Autodesk Fusion 360 part; units mm, degrees
note: some values were not read from the file. Set by a fixed rule: which sketch regions a step uses.
(part 41 of 59)
  spline S42 degree 5 poles (10.9662, -14.3955) (10.9662, -14.3956) (10.9663, -14.3958) (10.9664, -14.3961) (10.9666, -14.3966) (10.9669, -14.3973) (10.9672, -14.3981) (10.9676, -14.399) (10.9681, -14.4) (10.9685, -14.4011) (10.9691, -14.4023) (10.9696, -14.4036) (10.9702, -14.405) (10.9709, -14.4065) (10.9716, -14.408) (10.9724, -14.4097) (10.9731, -14.4115) (10.974, -14.4134) (10.9749, -14.4153) (10.9758, -14.4173) (10.9768, -14.4195) (10.9778, -14.4217) (10.9788, -14.424) (10.9799, -14.4263) (10.9811, -14.4288) (10.9823, -14.4313) (10.9835, -14.4339) (10.9848, -14.4366) (10.9861, -14.4394) (10.9875, -14.4423) (10.9889, -14.4452) (10.9903, -14.4482) (10.9918, -14.4513) (10.9934, -14.4544) (10.9949, -14.4577) (10.9966, -14.461) (10.9982, -14.4643) (10.9999, -14.4678) (11.0017, -14.4713) (11.0035, -14.4748) (11.0053, -14.4785) (11.0072, -14.4822) (11.0091, -14.486) (11.0111, -14.4898) (11.0131, -14.4937) (11.0151, -14.4977) (11.0172, -14.5017) (11.0193, -14.5058) (11.0215, -14.51) (11.0237, -14.5142) (11.0259, -14.5185) (11.0282, -14.5228) (11.0306, -14.5272) (11.0329, -14.5317) (11.0353, -14.5362) (11.0378, -14.5408) (11.0403, -14.5454) (11.0428, -14.5501) (11.0454, -14.5549) (11.048, -14.5597) (11.0507, -14.5645) (11.0534, -14.5694) (11.0561, -14.5744) (11.0589, -14.5794) (11.0617, -14.5845) (11.0646, -14.5896) (11.0675, -14.5948) (11.0704, -14.6) (11.0734, -14.6053) (11.0764, -14.6106) (11.0795, -14.616) (11.0826, -14.6214) (11.0857, -14.6269) (11.0889, -14.6324) (11.0921, -14.638) (11.0954, -14.6436) (11.0987, -14.6493) (11.102, -14.655) (11.1054, -14.6608) (11.1088, -14.6666) (11.1123, -14.6725) (11.1158, -14.6784) (11.1193, -14.6843) (11.1229, -14.6903) (11.1265, -14.6963) (11.1301, -14.7024) (11.1338, -14.7085) (11.1376, -14.7147) (11.1413, -14.7209) (11.1451, -14.7271) (11.149, -14.7334) (11.1529, -14.7397) (11.1568, -14.7461) (11.1608, -14.7525) (11.1648, -14.759) (11.1688, -14.7654) (11.1729, -14.772) (11.177, -14.7785) (11.1812, -14.7851) (11.1854, -14.7918) (11.1896, -14.7985) (11.1939, -14.8052) (11.1982, -14.8119) (11.2025, -14.8187) (11.2069, -14.8256) (11.2113, -14.8324) (11.2158, -14.8393) (11.2203, -14.8463) (11.2248, -14.8533) (11.2294, -14.8603) (11.234, -14.8673) (11.2387, -14.8744) (11.2434, -14.8815) (11.2481, -14.8887) (11.2529, -14.8958) (11.2577, -14.9031) (11.2625, -14.9103) (11.2674, -14.9176) (11.2723, -14.9249) (11.2773, -14.9323) (11.2823, -14.9396) (11.2873, -14.947) (11.2924, -14.9545) (11.2975, -14.962) (11.3026, -14.9695) (11.3078, -14.977) (11.313, -14.9846) (11.3183, -14.9922) (11.3235, -14.9998) (11.3289, -15.0074) (11.3342, -15.0151) (11.3396, -15.0228) (11.3451, -15.0306) (11.3506, -15.0384) (11.3561, -15.0462) (11.3616, -15.054) (11.3672, -15.0618) (11.3728, -15.0697) (11.3785, -15.0776) (11.3842, -15.0856) (11.3899, -15.0936) (11.3957, -15.1015) (11.4015, -15.1096) (11.4074, -15.1176) (11.4132, -15.1257) (11.4192, -15.1338) (11.4251, -15.1419) (11.4311, -15.1501) (11.4371, -15.1582) (11.4432, -15.1665) (11.4493, -15.1747) (11.4554, -15.1829) (11.4616, -15.1912) (11.4678, -15.1995) (11.4741, -15.2078) (11.4803, -15.2162) (11.4867, -15.2246) (11.493, -15.233) (11.4994, -15.2414) (11.5058, -15.2498) (11.5123, -15.2583) (11.5188, -15.2668) (11.5253, -15.2753) (11.5319, -15.2838) (11.5385, -15.2924) (11.5452, -15.301) (11.5518, -15.3096) (11.5585, -15.3182) (11.5653, -15.3268) (11.5721, -15.3355) (11.5789, -15.3442) (11.5858, -15.3529) (11.5927, -15.3616) (11.5996, -15.3704) (11.6065, -15.3791) (11.6135, -15.3879) (11.6206, -15.3967) (11.6276, -15.4055) (11.6348, -15.4144) (11.6419, -15.4233) (11.6491, -15.4322) (11.6563, -15.4411) (11.6635, -15.45) (11.6708, -15.4589) (11.6781, -15.4679) (11.6855, -15.4769) (11.6929, -15.4859) (11.7003, -15.4949) (11.7078, -15.5039) (11.7153, -15.513) (11.7228, -15.5221) (11.7303, -15.5312) (11.7379, -15.5403) (11.7456, -15.5494) (11.7532, -15.5585) (11.7609, -15.5677) (11.7687, -15.5769) (11.7765, -15.5861) (11.7843, -15.5953) (11.7921, -15.6045) (11.8, -15.6137) (11.8079, -15.623) (11.8158, -15.6323) (11.8238, -15.6416) (11.8318, -15.6509) (11.8399, -15.6602) (11.848, -15.6695) (11.8561, -15.6789) (11.8643, -15.6882) (11.8724, -15.6976) (11.8807, -15.707) (11.8889, -15.7164) (11.8972, -15.7259) (11.9055, -15.7353) (11.9139, -15.7447) (11.9223, -15.7542) (11.9307, -15.7637) (11.9392, -15.7732) (11.9477, -15.7827) (11.9562, -15.7922) (11.9648, -15.8018) (11.9734, -15.8113) (11.982, -15.8209) (11.9907, -15.8305) (11.9994, -15.84) (12.0081, -15.8496) (12.0169, -15.8593) (12.0257, -15.8689) (12.0345, -15.8785) (12.0434, -15.8882) (12.0523, -15.8978) (12.0613, -15.9075) (12.0702, -15.9172) (12.0792, -15.9269) (12.0883, -15.9366) (12.0973, -15.9464) (12.1065, -15.9561) (12.1156, -15.9658) (12.1248, -15.9756) (12.134, -15.9854) (12.1432, -15.9951) (12.1506, -16.003) (12.1562, -16.0089) (12.16, -16.0128) (12.1618, -16.0147) knots 0 0 0 0 0 0 0.00416667 0.00833333 0.0125 0.01666667 0.02083333 0.025 0.02916667 0.03333333 0.0375 0.04166667 0.04583333 0.05 0.05416667 0.05833333 0.0625 0.06666667 0.07083333 0.075 0.07916667 0.08333333 0.0875 0.09166667 0.09583333 0.1 0.10416667 0.10833333 0.1125 0.11666667 0.12083333 0.125 0.12916667 0.13333333 0.1375 0.14166667 0.14583333 0.15 0.15416667 0.15833333 0.1625 0.16666667 0.17083333 0.175 0.17916667 0.18333333 0.1875 0.19166667 0.19583333 0.2 0.20416667 0.20833333 0.2125 0.21666667 0.22083333 0.225 0.22916667 0.23333333 0.2375 0.24166667 0.24583333 0.25 0.25416667 0.25833333 0.2625 0.26666667 0.27083333 0.275 0.27916667 0.28333333 0.2875 0.29166667 0.29583333 0.3 0.30416667 0.30833333 0.3125 0.31666667 0.32083333 0.325 0.32916667 0.33333333 0.3375 0.34166667 0.34583333 0.35 0.35416667 0.35833333 0.3625 0.36666667 0.37083333 0.375 0.37916667 0.38333333 0.3875 0.39166667 0.39583333 0.4 0.40416667 0.40833333 0.4125 0.41666667 0.42083333 0.425 0.42916667 0.43333333 0.4375 0.44166667 0.44583333 0.45 0.45416667 0.45833333 0.4625 0.46666667 0.47083333 0.475 0.47916667 0.48333333 0.4875 0.49166667 0.49583333 0.5 0.50416667 0.50833333 0.5125 0.51666667 0.52083333 0.525 0.52916667 0.53333333 0.5375 0.54166667 0.54583333 0.55 0.55416667 0.55833333 0.5625 0.56666667 0.57083333 0.575 0.57916667 0.58333333 0.5875 0.59166667 0.59583333 0.6 0.60416667 0.60833333 0.6125 0.61666667 0.62083333 0.625 0.62916667 0.63333333 0.6375 0.64166667 0.64583333 0.65 0.65416667 0.65833333 0.6625 0.66666667 0.67083333 0.675 0.67916667 0.68333333 0.6875 0.69166667 0.69583333 0.7 0.70416667 0.70833333 0.7125 0.71666667 0.72083333 0.725 0.72916667 0.73333333 0.7375 0.74166667 0.74583333 0.75 0.75416667 0.75833333 0.7625 0.76666667 0.77083333 0.775 0.77916667 0.78333333 0.7875 0.79166667 0.79583333 0.8 0.80416667 0.80833333 0.8125 0.81666667 0.82083333 0.825 0.82916667 0.83333333 0.8375 0.84166667 0.84583333 0.85 0.85416667 0.85833333 0.8625 0.86666667 0.87083333 0.875 0.87916667 0.88333333 0.8875 0.89166667 0.89583333 0.9 0.90416667 0.90833333 0.9125 0.91666667 0.92083333 0.925 0.92916667 0.93333333 0.9375 0.94166667 0.94583333 0.95 0.95416667 0.95833333 0.9625 0.96666667 0.97083333 0.975 0.97916667 0.98333333 0.9875 0.99166667 0.99583333 1 1 1 1 1 1
  arc A43 (12.1618, -16.0147) -> (13.0527, -15.6181) centre (0, 12.5) ccw
  spline S43 degree 5 poles (13.0527, -15.6181) (13.0525, -15.6154) (13.0521, -15.61) (13.0515, -15.6019) (13.0506, -15.5911) (13.0495, -15.5777) (13.0484, -15.5644) (13.0473, -15.551) (13.0462, -15.5377) (13.0451, -15.5244) (13.0439, -15.5112) (13.0427, -15.4979) (13.0415, -15.4848) (13.0404, -15.4716) (13.0391, -15.4585) (13.0379, -15.4454) (13.0367, -15.4323) (13.0354, -15.4193) (13.0342, -15.4063) (13.0329, -15.3934) (13.0316, -15.3805) (13.0303, -15.3676) (13.029, -15.3547) (13.0276, -15.3419) (13.0263, -15.3291) (13.0249, -15.3164) (13.0236, -15.3037) (13.0222, -15.291) (13.0208, -15.2784) (13.0194, -15.2658) (13.018, -15.2532) (13.0165, -15.2406) (13.0151, -15.2281) (13.0136, -15.2157) (13.0122, -15.2032) (13.0107, -15.1908) (13.0092, -15.1785) (13.0077, -15.1661) (13.0062, -15.1539) (13.0047, -15.1416) (13.0031, -15.1294) (13.0016, -15.1172) (13, -15.105) (12.9984, -15.0929) (12.9968, -15.0809) (12.9952, -15.0688) (12.9936, -15.0568) (12.992, -15.0449) (12.9904, -15.0329) (12.9887, -15.021) (12.9871, -15.0092) (12.9854, -14.9974) (12.9838, -14.9856) (12.9821, -14.9738) (12.9804, -14.9621) (12.9787, -14.9505) (12.977, -14.9388) (12.9752, -14.9273) (12.9735, -14.9157) (12.9718, -14.9042) (12.97, -14.8927) (12.9682, -14.8813) (12.9665, -14.8699) (12.9647, -14.8585) (12.9629, -14.8472) (12.9611, -14.8359) (12.9593, -14.8247) (12.9574, -14.8135) (12.9556, -14.8023) (12.9538, -14.7912) (12.9519, -14.7801) (12.9501, -14.7691) (12.9482, -14.7581) (12.9463, -14.7471) (12.9445, -14.7362) (12.9426, -14.7253) (12.9407, -14.7145) (12.9388, -14.7037) (12.9368, -14.6929) (12.9349, -14.6822) (12.933, -14.6715) (12.9311, -14.6609) (12.9291, -14.6503) (12.9272, -14.6397) (12.9252, -14.6292) (12.9232, -14.6188) (12.9213, -14.6083) (12.9193, -14.5979) (12.9173, -14.5876) (12.9153, -14.5773) (12.9133, -14.5671) (12.9113, -14.5568) (12.9093, -14.5467) (12.9072, -14.5365) (12.9052, -14.5265) (12.9032, -14.5164) (12.9011, -14.5064) (12.8991, -14.4965) (12.8971, -14.4866) (12.895, -14.4767) (12.8929, -14.4669) (12.8909, -14.4571) (12.8888, -14.4474) (12.8867, -14.4377) (12.8847, -14.4281) (12.8826, -14.4185) (12.8805, -14.4089) (12.8784, -14.3994) (12.8763, -14.39) (12.8742, -14.3806) (12.8721, -14.3712) (12.87, -14.3619) (12.8679, -14.3526) (12.8658, -14.3434) (12.8636, -14.3342) (12.8615, -14.3251) (12.8594, -14.316) (12.8573, -14.3069) (12.8551, -14.298) (12.853, -14.289) (12.8509, -14.2801) (12.8487, -14.2713) (12.8466, -14.2625) (12.8445, -14.2537) (12.8423, -14.2451) (12.8402, -14.2364) (12.838, -14.2278) (12.8359, -14.2193) (12.8337, -14.2108) (12.8316, -14.2023) (12.8294, -14.1939) (12.8273, -14.1856) (12.8251, -14.1773) (12.823, -14.169) (12.8208, -14.1608) (12.8187, -14.1527) (12.8166, -14.1446) (12.8144, -14.1365) (12.8123, -14.1286) (12.8101, -14.1206) (12.808, -14.1127) (12.8058, -14.1049) (12.8037, -14.0971) (12.8016, -14.0894) (12.7994, -14.0817) (12.7973, -14.0741) (12.7952, -14.0665) (12.793, -14.059) (12.7909, -14.0516) (12.7888, -14.0442) (12.7867, -14.0368) (12.7845, -14.0296) (12.7824, -14.0223) (12.7803, -14.0151) (12.7782, -14.008) (12.7761, -14.0009) (12.774, -13.9939) (12.772, -13.987) (12.7699, -13.9801) (12.7678, -13.9733) (12.7657, -13.9665) (12.7637, -13.9598) (12.7616, -13.9531) (12.7596, -13.9465) (12.7575, -13.9399) (12.7555, -13.9335) (12.7534, -13.927) (12.7514, -13.9207) (12.7494, -13.9144) (12.7474, -13.9081) (12.7454, -13.9019) (12.7434, -13.8958) (12.7414, -13.8897) (12.7395, -13.8837) (12.7375, -13.8778) (12.7356, -13.8719) (12.7336, -13.8661) (12.7317, -13.8604) (12.7298, -13.8547) (12.7279, -13.8491) (12.726, -13.8435) (12.7241, -13.838) (12.7222, -13.8326) (12.7204, -13.8273) (12.7185, -13.822) (12.7167, -13.8167) (12.7149, -13.8116) (12.7131, -13.8065) (12.7113, -13.8015) (12.7095, -13.7965) (12.7077, -13.7916) (12.706, -13.7868) (12.7043, -13.782) (12.7026, -13.7774) (12.7009, -13.7728) (12.6992, -13.7682) (12.6975, -13.7638) (12.6959, -13.7594) (12.6943, -13.755) (12.6927, -13.7508) (12.6911, -13.7466) (12.6895, -13.7425) (12.688, -13.7385) (12.6864, -13.7345) (12.6849, -13.7307) (12.6834, -13.7269) (12.682, -13.7231) (12.6806, -13.7195) (12.6791, -13.7159) (12.6778, -13.7124) (12.6764, -13.709) (12.675, -13.7057) (12.6737, -13.7024) (12.6724, -13.6993) (12.6712, -13.6962) (12.6699, -13.6932) (12.6687, -13.6903) (12.6676, -13.6874) (12.6664, -13.6847) (12.6653, -13.682) (12.6642, -13.6794) (12.6631, -13.6769) (12.6621, -13.6745) (12.6611, -13.6722) (12.6602, -13.67) (12.6592, -13.6678) (12.6583, -13.6658) (12.6575, -13.6638) (12.6567, -13.6619) (12.6559, -13.6602) (12.6551, -13.6585) (12.6544, -13.6569) (12.6538, -13.6554) (12.6531, -13.654) (12.6526, -13.6527) (12.652, -13.6515) (12.6515, -13.6504) (12.651, -13.6495) (12.6506, -13.6486) (12.6503, -13.6478) (12.65, -13.6471) (12.6497, -13.6467) (12.6496, -13.6464) (12.6495, -13.6462) (12.6495, -13.6461) knots -1 -1 -1 -1 -1 -1 -0.99583333 -0.99166667 -0.9875 -0.98333333 -0.97916667 -0.975 -0.97083333 -0.96666667 -0.9625 -0.95833333 -0.95416667 -0.95 -0.94583333 -0.94166667 -0.9375 -0.93333333 -0.92916667 -0.925 -0.92083333 -0.91666667 -0.9125 -0.90833333 -0.90416667 -0.9 -0.89583333 -0.89166667 -0.8875 -0.88333333 -0.87916667 -0.875 -0.87083333 -0.86666667 -0.8625 -0.85833333 -0.85416667 -0.85 -0.84583333 -0.84166667 -0.8375 -0.83333333 -0.82916667 -0.825 -0.82083333 -0.81666667 -0.8125 -0.80833333 -0.80416667 -0.8 -0.79583333 -0.79166667 -0.7875 -0.78333333 -0.77916667 -0.775 -0.77083333 -0.76666667 -0.7625 -0.75833333 -0.75416667 -0.75 -0.74583333 -0.74166667 -0.7375 -0.73333333 -0.72916667 -0.725 -0.72083333 -0.71666667 -0.7125 -0.70833333 -0.70416667 -0.7 -0.69583333 -0.69166667 -0.6875 -0.68333333 -0.67916667 -0.675 -0.67083333 -0.66666667 -0.6625 -0.65833333 -0.65416667 -0.65 -0.64583333 -0.64166667 -0.6375 -0.63333333 -0.62916667 -0.625 -0.62083333 -0.61666667 -0.6125 -0.60833333 -0.60416667 -0.6 -0.59583333 -0.59166667 -0.5875 -0.58333333 -0.57916667 -0.575 -0.57083333 -0.56666667 -0.5625 -0.55833333 -0.55416667 -0.55 -0.54583333 -0.54166667 -0.5375 -0.53333333 -0.52916667 -0.525 -0.52083333 -0.51666667 -0.5125 -0.50833333 -0.50416667 -0.5 -0.49583333 -0.49166667 -0.4875 -0.48333333 -0.47916667 -0.475 -0.47083333 -0.46666667 -0.4625 -0.45833333 -0.45416667 -0.45 -0.44583333 -0.44166667 -0.4375 -0.43333333 -0.42916667 -0.425 -0.42083333 -0.41666667 -0.4125 -0.40833333 -0.40416667 -0.4 -0.39583333 -0.39166667 -0.3875 -0.38333333 -0.37916667 -0.375 -0.37083333 -0.36666667 -0.3625 -0.35833333 -0.35416667 -0.35 -0.34583333 -0.34166667 -0.3375 -0.33333333 -0.32916667 -0.325 -0.32083333 -0.31666667 -0.3125 -0.30833333 -0.30416667 -0.3 -0.29583333 -0.29166667 -0.2875 -0.28333333 -0.27916667 -0.275 -0.27083333 -0.26666667 -0.2625 -0.25833333 -0.25416667 -0.25 -0.24583333 -0.24166667 -0.2375 -0.23333333 -0.22916667 -0.225 -0.22083333 -0.21666667 -0.2125 -0.20833333 -0.20416667 -0.2 -0.19583333 -0.19166667 -0.1875 -0.18333333 -0.17916667 -0.175 -0.17083333 -0.16666667 -0.1625 -0.15833333 -0.15416667 -0.15 -0.14583333 -0.14166667 -0.1375 -0.13333333 -0.12916667 -0.125 -0.12083333 -0.11666667 -0.1125 -0.10833333 -0.10416667 -0.1 -0.09583333 -0.09166667 -0.0875 -0.08333333 -0.07916667 -0.075 -0.07083333 -0.06666667 -0.0625 -0.05833333 -0.05416667 -0.05 -0.04583333 -0.04166667 -0.0375 -0.03333333 -0.02916667 -0.025 -0.02083333 -0.01666667 -0.0125 -0.00833333 -0.00416667 0 0 0 0 0 0
  line L95 (12.6495, -13.6461) -> (12.6491, -13.6453)
  line L96 (12.6491, -13.6453) -> (12.5209, -13.3803)
  arc A44 (12.5209, -13.3803) -> (13.578, -12.8417) centre (0, 12.5) ccw
  line L97 (13.578, -12.8417) -> (13.7171, -13.1012)
  line L98 (13.7171, -13.1012) -> (13.7175, -13.1019)
  spline S44 degree 5 poles (13.7175, -13.1019) (13.7175, -13.102) (13.7176, -13.1022) (13.7178, -13.1025) (13.718, -13.1029) (13.7184, -13.1036) (13.7188, -13.1043) (13.7193, -13.1052) (13.7198, -13.1061) (13.7204, -13.1072) (13.721, -13.1083) (13.7217, -13.1096) (13.7225, -13.1109) (13.7233, -13.1123) (13.7242, -13.1138) (13.7251, -13.1154) (13.7261, -13.1171) (13.7271, -13.1188) (13.7282, -13.1207) (13.7293, -13.1226) (13.7305, -13.1246) (13.7317, -13.1267) (13.733, -13.1289) (13.7344, -13.1311) (13.7358, -13.1334) (13.7372, -13.1358) (13.7387, -13.1383) (13.7403, -13.1409) (13.7419, -13.1435) (13.7435, -13.1462) (13.7452, -13.1489) (13.747, -13.1518) (13.7488, -13.1547) (13.7506, -13.1577) (13.7526, -13.1607) (13.7545, -13.1638) (13.7565, -13.167) (13.7586, -13.1702) (13.7607, -13.1735) (13.7628, -13.1769) (13.765, -13.1803) (13.7673, -13.1838) (13.7696, -13.1874) (13.7719, -13.191) (13.7743, -13.1947) (13.7768, -13.1984) (13.7793, -13.2022) (13.7818, -13.206) (13.7844, -13.21) (13.787, -13.2139) (13.7897, -13.218) (13.7925, -13.222) (13.7952, -13.2262) (13.7981, -13.2304) (13.8009, -13.2346) (13.8039, -13.2389) (13.8068, -13.2432) (13.8098, -13.2476) (13.8129, -13.2521) (13.816, -13.2566) (13.8192, -13.2612) (13.8224, -13.2658) (13.8256, -13.2704) (13.8289, -13.2751) (13.8322, -13.2799) (13.8356, -13.2847) (13.839, -13.2895) (13.8425, -13.2944) (13.846, -13.2993) (13.8496, -13.3043) (13.8532, -13.3093) (13.8568, -13.3144) (13.8605, -13.3195) (13.8643, -13.3247) (13.8681, -13.3299) (13.8719, -13.3352) (13.8758, -13.3405) (13.8797, -13.3458) (13.8836, -13.3512) (13.8876, -13.3566) (13.8917, -13.3621) (13.8958, -13.3676) (13.8999, -13.3731) (13.9041, -13.3787) (13.9083, -13.3843) (13.9126, -13.39) (13.9169, -13.3957) (13.9213, -13.4014) (13.9257, -13.4072) (13.9301, -13.413) (13.9346, -13.4188) (13.9391, -13.4247) (13.9437, -13.4306) (13.9483, -13.4366) (13.9529, -13.4426) (13.9576, -13.4486) (13.9624, -13.4547) (13.9672, -13.4608) (13.972, -13.4669) (13.9769, -13.4731) (13.9818, -13.4793) (13.9867, -13.4855) (13.9917, -13.4918) (13.9967, -13.4981) (14.0018, -13.5044) (14.0069, -13.5108) (14.0121, -13.5172) (14.0173, -13.5236) (14.0225, -13.5301) (14.0278, -13.5366) (14.0332, -13.5431) (14.0385, -13.5497) (14.0439, -13.5563) (14.0494, -13.5629) (14.0549, -13.5695) (14.0604, -13.5762) (14.066, -13.5829) (14.0716, -13.5896) (14.0772, -13.5964) (14.0829, -13.6032) (14.0887, -13.61) (14.0945, -13.6168) (14.1003, -13.6237) (14.1061, -13.6306) (14.112, -13.6375) (14.118, -13.6445) (14.1239, -13.6515) (14.13, -13.6585) (14.136, -13.6655) (14.1421, -13.6726) (14.1483, -13.6796) (14.1544, -13.6868) (14.1607, -13.6939) (14.1669, -13.701) (14.1732, -13.7082) (14.1796, -13.7154) (14.1859, -13.7227) (14.1924, -13.7299) (14.1988, -13.7372) (14.2053, -13.7445) (14.2119, -13.7518) (14.2184, -13.7592) (14.225, -13.7665) (14.2317, -13.7739) (14.2384, -13.7813) (14.2451, -13.7888) (14.2519, -13.7962) (14.2587, -13.8037) (14.2656, -13.8112) (14.2724, -13.8188) (14.2794, -13.8263) (14.2863, -13.8339) (14.2933, -13.8414) (14.3004, -13.8491) (14.3075, -13.8567) (14.3146, -13.8643) (14.3217, -13.872) (14.3289, -13.8797) (14.3362, -13.8874) (14.3435, -13.8951) (14.3508, -13.9029) (14.3581, -13.9106) (14.3655, -13.9184) (14.3729, -13.9262) (14.3804, -13.934) (14.3879, -13.9419) (14.3954, -13.9497) (14.403, -13.9576) (14.4106, -13.9655) (14.4183, -13.9734) (14.426, -13.9813) (14.4337, -13.9893) (14.4415, -13.9972) (14.4493, -14.0052) (14.4571, -14.0132) (14.465, -14.0212) (14.4729, -14.0292) (14.4809, -14.0373) (14.4889, -14.0453) (14.4969, -14.0534) (14.505, -14.0615) (14.5131, -14.0696) (14.5212, -14.0777) (14.5294, -14.0858) (14.5376, -14.094) (14.5459, -14.1022) (14.5541, -14.1103) (14.5625, -14.1185) (14.5708, -14.1267) (14.5792, -14.135) (14.5877, -14.1432) (14.5961, -14.1514) (14.6046, -14.1597) (14.6132, -14.168) (14.6218, -14.1763) (14.6304, -14.1846) (14.639, -14.1929) (14.6477, -14.2012) (14.6565, -14.2096) (14.6652, -14.2179) (14.674, -14.2263) (14.6829, -14.2347) (14.6917, -14.2431) (14.7006, -14.2515) (14.7096, -14.2599) (14.7186, -14.2683) (14.7276, -14.2767) (14.7366, -14.2852) (14.7457, -14.2937) (14.7549, -14.3021) (14.764, -14.3106) (14.7732, -14.3191) (14.7824, -14.3276) (14.7917, -14.3361) (14.801, -14.3447) (14.8104, -14.3532) (14.8197, -14.3618) (14.8291, -14.3703) (14.8386, -14.3789) (14.8481, -14.3875) (14.8576, -14.3961) (14.8671, -14.4047) (14.8767, -14.4133) (14.8863, -14.4219) (14.896, -14.4305) (14.9057, -14.4392) (14.9154, -14.4478) (14.9252, -14.4565) (14.935, -14.4651) (14.9448, -14.4738) (14.9547, -14.4825) (14.9646, -14.4912) (14.9745, -14.4999) (14.9845, -14.5086) (14.9945, -14.5173) (15.0045, -14.526) (15.0146, -14.5347) (15.0247, -14.5435) (15.0349, -14.5522) (15.045, -14.561) (15.0553, -14.5697) (15.0635, -14.5767) (15.0696, -14.582) (15.0737, -14.5855) (15.0758, -14.5873) knots 0 0 0 0 0 0 0.00416667 0.00833333 0.0125 0.01666667 0.02083333 0.025 0.02916667 0.03333333 0.0375 0.04166667 0.04583333 0.05 0.05416667 0.05833333 0.0625 0.06666667 0.07083333 0.075 0.07916667 0.08333333 0.0875 0.09166667 0.09583333 0.1 0.10416667 0.10833333 0.1125 0.11666667 0.12083333 0.125 0.12916667 0.13333333 0.1375 0.14166667 0.14583333 0.15 0.15416667 0.15833333 0.1625 0.16666667 0.17083333 0.175 0.17916667 0.18333333 0.1875 0.19166667 0.19583333 0.2 0.20416667 0.20833333 0.2125 0.21666667 0.22083333 0.225 0.22916667 0.23333333 0.2375 0.24166667 0.24583333 0.25 0.25416667 0.25833333 0.2625 0.26666667 0.27083333 0.275 0.27916667 0.28333333 0.2875 0.29166667 0.29583333 0.3 0.30416667 0.30833333 0.3125 0.31666667 0.32083333 0.325 0.32916667 0.33333333 0.3375 0.34166667 0.34583333 0.35 0.35416667 0.35833333 0.3625 0.36666667 0.37083333 0.375 0.37916667 0.38333333 0.3875 0.39166667 0.39583333 0.4 0.40416667 0.40833333 0.4125 0.41666667 0.42083333 0.425 0.42916667 0.43333333 0.4375 0.44166667 0.44583333 0.45 0.45416667 0.45833333 0.4625 0.46666667 0.47083333 0.475 0.47916667 0.48333333 0.4875 0.49166667 0.49583333 0.5 0.50416667 0.50833333 0.5125 0.51666667 0.52083333 0.525 0.52916667 0.53333333 0.5375 0.54166667 0.54583333 0.55 0.55416667 0.55833333 0.5625 0.56666667 0.57083333 0.575 0.57916667 0.58333333 0.5875 0.59166667 0.59583333 0.6 0.60416667 0.60833333 0.6125 0.61666667 0.62083333 0.625 0.62916667 0.63333333 0.6375 0.64166667 0.64583333 0.65 0.65416667 0.65833333 0.6625 0.66666667 0.67083333 0.675 0.67916667 0.68333333 0.6875 0.69166667 0.69583333 0.7 0.70416667 0.70833333 0.7125 0.71666667 0.72083333 0.725 0.72916667 0.73333333 0.7375 0.74166667 0.74583333 0.75 0.75416667 0.75833333 0.7625 0.76666667 0.77083333 0.775 0.77916667 0.78333333 0.7875 0.79166667 0.79583333 0.8 0.80416667 0.80833333 0.8125 0.81666667 0.82083333 0.825 0.82916667 0.83333333 0.8375 0.84166667 0.84583333 0.85 0.85416667 0.85833333 0.8625 0.86666667 0.87083333 0.875 0.87916667 0.88333333 0.8875 0.89166667 0.89583333 0.9 0.90416667 0.90833333 0.9125 0.91666667 0.92083333 0.925 0.92916667 0.93333333 0.9375 0.94166667 0.94583333 0.95 0.95416667 0.95833333 0.9625 0.96666667 0.97083333 0.975 0.97916667 0.98333333 0.9875 0.99166667 0.99583333 1 1 1 1 1 1
  arc A45 (15.0758, -14.5873) -> (15.9204, -14.0997) centre (0, 12.5) ccw
  spline S45 degree 5 poles (15.9204, -14.0997) (15.9199, -14.097) (15.9189, -14.0917) (15.9174, -14.0837) (15.9154, -14.0731) (15.913, -14.0599) (15.9105, -14.0467) (15.908, -14.0335) (15.9055, -14.0204) (15.9029, -14.0073) (15.9004, -13.9943) (15.8979, -13.9812) (15.8953, -13.9682) (15.8927, -13.9553) (15.8902, -13.9424) (15.8876, -13.9295) (15.885, -13.9166) (15.8824, -13.9038) (15.8798, -13.891) (15.8771, -13.8783) (15.8745, -13.8656) (15.8719, -13.8529) (15.8692, -13.8403) (15.8666, -13.8276) (15.8639, -13.8151) (15.8612, -13.8025) (15.8585, -13.79) (15.8558, -13.7776) (15.8531, -13.7651) (15.8504, -13.7528) (15.8477, -13.7404) (15.8449, -13.7281) (15.8422, -13.7158) (15.8394, -13.7035) (15.8367, -13.6913) (15.8339, -13.6792) (15.8311, -13.667) (15.8283, -13.6549) (15.8255, -13.6428) (15.8227, -13.6308) (15.8199, -13.6188) (15.8171, -13.6069) (15.8143, -13.595) (15.8115, -13.5831) (15.8086, -13.5712) (15.8058, -13.5594) (15.8029, -13.5477) (15.8001, -13.5359) (15.7972, -13.5242) (15.7943, -13.5126) (15.7914, -13.501) (15.7886, -13.4894) (15.7857, -13.4778) (15.7828, -13.4663) (15.7798, -13.4549) (15.7769, -13.4435) (15.774, -13.4321) (15.7711, -13.4207) (15.7682, -13.4094) (15.7652, -13.3982) (15.7623, -13.3869) (15.7593, -13.3757) (15.7564, -13.3646) (15.7534, -13.3535) (15.7504, -13.3424) (15.7475, -13.3314) (15.7445, -13.3204) (15.7415, -13.3094) (15.7385, -13.2985) (15.7355, -13.2877) (15.7325, -13.2768) (15.7295, -13.266) (15.7265, -13.2553) (15.7235, -13.2446) (15.7205, -13.2339) (15.7175, -13.2233) (15.7145, -13.2127) (15.7114, -13.2022) (15.7084, -13.1917) (15.7054, -13.1812) (15.7023, -13.1708) (15.6993, -13.1604) (15.6963, -13.1501) (15.6932, -13.1398) (15.6902, -13.1296) (15.6871, -13.1194) (15.6841, -13.1092) (15.681, -13.0991) (15.6779, -13.089) (15.6749, -13.079) (15.6718, -13.069) (15.6688, -13.059) (15.6657, -13.0491) (15.6626, -13.0393) (15.6596, -13.0294) (15.6565, -13.0197) (15.6534, -13.0099) (15.6503, -13.0003) (15.6473, -12.9906) (15.6442, -12.981) (15.6411, -12.9715) (15.638, -12.962) (15.635, -12.9525) (15.6319, -12.9431) (15.6288, -12.9337) (15.6257, -12.9244) (15.6227, -12.9151) (15.6196, -12.9059) (15.6165, -12.8967) (15.6134, -12.8876) (15.6104, -12.8785) (15.6073, -12.8694) (15.6042, -12.8604) (15.6012, -12.8515) (15.5981, -12.8426) (15.595, -12.8337) (15.592, -12.8249) (15.5889, -12.8161) (15.5859, -12.8074) (15.5828, -12.7988) (15.5798, -12.7901) (15.5767, -12.7816) (15.5737, -12.7731) (15.5706, -12.7646) (15.5676, -12.7562) (15.5645, -12.7478) (15.5615, -12.7394) (15.5585, -12.7312) (15.5555, -12.7229) (15.5524, -12.7148) (15.5494, -12.7066) (15.5464, -12.6986) (15.5434, -12.6905) (15.5404, -12.6826) (15.5374, -12.6746) (15.5344, -12.6668) (15.5315, -12.6589) (15.5285, -12.6512) (15.5255, -12.6434) (15.5226, -12.6358) (15.5196, -12.6282) (15.5166, -12.6206) (15.5137, -12.6131) (15.5108, -12.6056) (15.5078, -12.5982) (15.5049, -12.5909) (15.502, -12.5836) (15.4991, -12.5763) (15.4962, -12.5691) (15.4933, -12.562) (15.4905, -12.5549) (15.4876, -12.5479) (15.4848, -12.5409) (15.4819, -12.534) (15.4791, -12.5271) (15.4762, -12.5203) (15.4734, -12.5136) (15.4706, -12.5069) (15.4678, -12.5002) (15.4651, -12.4936) (15.4623, -12.4871) (15.4595, -12.4806) (15.4568, -12.4742) (15.4541, -12.4679) (15.4514, -12.4616) (15.4486, -12.4553) (15.446, -12.4492) (15.4433, -12.443) (15.4406, -12.437) (15.438, -12.431) (15.4353, -12.425) (15.4327, -12.4192) (15.4301, -12.4133) (15.4275, -12.4076) (15.425, -12.4019) (15.4224, -12.3962) (15.4199, -12.3907) (15.4174, -12.3852) (15.4149, -12.3797) (15.4124, -12.3743) (15.4099, -12.369) (15.4075, -12.3637) (15.405, -12.3585) (15.4026, -12.3534) (15.4002, -12.3483) (15.3979, -12.3433) (15.3955, -12.3384) (15.3932, -12.3335) (15.3909, -12.3287) (15.3886, -12.3239) (15.3863, -12.3193) (15.3841, -12.3147) (15.3819, -12.3101) (15.3797, -12.3056) (15.3775, -12.3012) (15.3754, -12.2969) (15.3733, -12.2926) (15.3712, -12.2884) (15.3691, -12.2843) (15.3671, -12.2802) (15.3651, -12.2763) (15.3631, -12.2723) (15.3611, -12.2685) (15.3592, -12.2647) (15.3573, -12.261) (15.3554, -12.2574) (15.3536, -12.2539) (15.3518, -12.2504) (15.35, -12.247) (15.3482, -12.2437) (15.3465, -12.2404) (15.3449, -12.2372) (15.3432, -12.2341) (15.3416, -12.2311) (15.34, -12.2282) (15.3385, -12.2253) (15.337, -12.2225) (15.3355, -12.2198) (15.3341, -12.2172) (15.3327, -12.2147) (15.3313, -12.2122) (15.33, -12.2099) (15.3287, -12.2076) (15.3275, -12.2054) (15.3263, -12.2033) (15.3252, -12.2012) (15.3241, -12.1993) (15.323, -12.1974) (15.322, -12.1956) (15.321, -12.194) (15.3201, -12.1924) (15.3193, -12.1909) (15.3184, -12.1895) (15.3177, -12.1881) (15.3169, -12.1869) (15.3163, -12.1858) (15.3157, -12.1848) (15.3151, -12.1838) (15.3146, -12.183) (15.3142, -12.1822) (15.3138, -12.1816) (15.3135, -12.1812) (15.3133, -12.1809) (15.3132, -12.1807) (15.3132, -12.1806) knots -1 -1 -1 -1 -1 -1 -0.99583333 -0.99166667 -0.9875 -0.98333333 -0.97916667 -0.975 -0.97083333 -0.96666667 -0.9625 -0.95833333 -0.95416667 -0.95 -0.94583333 -0.94166667 -0.9375 -0.93333333 -0.92916667 -0.925 -0.92083333 -0.91666667 -0.9125 -0.90833333 -0.90416667 -0.9 -0.89583333 -0.89166667 -0.8875 -0.88333333 -0.87916667 -0.875 -0.87083333 -0.86666667 -0.8625 -0.85833333 -0.85416667 -0.85 -0.84583333 -0.84166667 -0.8375 -0.83333333 -0.82916667 -0.825 -0.82083333 -0.81666667 -0.8125 -0.80833333 -0.80416667 -0.8 -0.79583333 -0.79166667 -0.7875 -0.78333333 -0.77916667 -0.775 -0.77083333 -0.76666667 -0.7625 -0.75833333 -0.75416667 -0.75 -0.74583333 -0.74166667 -0.7375 -0.73333333 -0.72916667 -0.725 -0.72083333 -0.71666667 -0.7125 -0.70833333 -0.70416667 -0.7 -0.69583333 -0.69166667 -0.6875 -0.68333333 -0.67916667 -0.675 -0.67083333 -0.66666667 -0.6625 -0.65833333 -0.65416667 -0.65 -0.64583333 -0.64166667 -0.6375 -0.63333333 -0.62916667 -0.625 -0.62083333 -0.61666667 -0.6125 -0.60833333 -0.60416667 -0.6 -0.59583333 -0.59166667 -0.5875 -0.58333333 -0.57916667 -0.575 -0.57083333 -0.56666667 -0.5625 -0.55833333 -0.55416667 -0.55 -0.54583333 -0.54166667 -0.5375 -0.53333333 -0.52916667 -0.525 -0.52083333 -0.51666667 -0.5125 -0.50833333 -0.50416667 -0.5 -0.49583333 -0.49166667 -0.4875 -0.48333333 -0.47916667 -0.475 -0.47083333 -0.46666667 -0.4625 -0.45833333 -0.45416667 -0.45 -0.44583333 -0.44166667 -0.4375 -0.43333333 -0.42916667 -0.425 -0.42083333 -0.41666667 -0.4125 -0.40833333 -0.40416667 -0.4 -0.39583333 -0.39166667 -0.3875 -0.38333333 -0.37916667 -0.375 -0.37083333 -0.36666667 -0.3625 -0.35833333 -0.35416667 -0.35 -0.34583333 -0.34166667 -0.3375 -0.33333333 -0.32916667 -0.325 -0.32083333 -0.31666667 -0.3125 -0.30833333 -0.30416667 -0.3 -0.29583333 -0.29166667 -0.2875 -0.28333333 -0.27916667 -0.275 -0.27083333 -0.26666667 -0.2625 -0.25833333 -0.25416667 -0.25 -0.24583333 -0.24166667 -0.2375 -0.23333333 -0.22916667 -0.225 -0.22083333 -0.21666667 -0.2125 -0.20833333 -0.20416667 -0.2 -0.19583333 -0.19166667 -0.1875 -0.18333333 -0.17916667 -0.175 -0.17083333 -0.16666667 -0.1625 -0.15833333 -0.15416667 -0.15 -0.14583333 -0.14166667 -0.1375 -0.13333333 -0.12916667 -0.125 -0.12083333 -0.11666667 -0.1125 -0.10833333 -0.10416667 -0.1 -0.09583333 -0.09166667 -0.0875 -0.08333333 -0.07916667 -0.075 -0.07083333 -0.06666667 -0.0625 -0.05833333 -0.05416667 -0.05 -0.04583333 -0.04166667 -0.0375 -0.03333333 -0.02916667 -0.025 -0.02083333 -0.01666667 -0.0125 -0.00833333 -0.00416667 0 0 0 0 0 0
  line L99 (15.3132, -12.1806) -> (15.3128, -12.1799)
  line L100 (15.3128, -12.1799) -> (15.1575, -11.9297)
  arc A46 (15.1575, -11.9297) -> (16.1526, -11.2836) centre (0, 12.5) ccw
  line L101 (16.1526, -11.2836) -> (16.318, -11.5271)
  line L102 (16.318, -11.5271) -> (16.3184, -11.5278)
  spline S46 degree 5 poles (16.3184, -11.5278) (16.3185, -11.5279) (16.3186, -11.5281) (16.3188, -11.5283) (16.3191, -11.5287) (16.3195, -11.5294) (16.32, -11.5301) (16.3206, -11.5309) (16.3212, -11.5317) (16.3219, -11.5327) (16.3227, -11.5338) (16.3235, -11.535) (16.3244, -11.5362) (16.3253, -11.5375) (16.3263, -11.5389) (16.3274, -11.5404) (16.3286, -11.542) (16.3298, -11.5436) (16.331, -11.5453) (16.3324, -11.5471) (16.3338, -11.549) (16.3352, -11.551) (16.3367, -11.553) (16.3383, -11.5551) (16.3399, -11.5572) (16.3416, -11.5595) (16.3434, -11.5618) (16.3452, -11.5641) (16.3471, -11.5666) (16.349, -11.5691) (16.351, -11.5717) (16.353, -11.5743) (16.3551, -11.577) (16.3573, -11.5798) (16.3595, -11.5826) (16.3618, -11.5855) (16.3641, -11.5884) (16.3665, -11.5914) (16.3689, -11.5945) (16.3714, -11.5976) (16.374, -11.6008) (16.3766, -11.604) (16.3792, -11.6073) (16.3819, -11.6107) (16.3847, -11.6141) (16.3875, -11.6176) (16.3904, -11.6211) (16.3933, -11.6246) (16.3963, -11.6283) (16.3994, -11.6319) (16.4024, -11.6356) (16.4056, -11.6394) (16.4088, -11.6432) (16.412, -11.6471) (16.4153, -11.651) (16.4187, -11.655) (16.4221, -11.659) (16.4256, -11.6631) (16.4291, -11.6672) (16.4326, -11.6713) (16.4362, -11.6755) (16.4399, -11.6798) (16.4436, -11.6841) (16.4474, -11.6884) (16.4512, -11.6928) (16.455, -11.6972) (16.459, -11.7017) (16.4629, -11.7062) (16.4669, -11.7107) (16.471, -11.7153) (16.4751, -11.7199) (16.4793, -11.7246) (16.4835, -11.7293) (16.4877, -11.734) (16.492, -11.7388) (16.4964, -11.7436) (16.5008, -11.7485) (16.5053, -11.7534) (16.5098, -11.7583) (16.5143, -11.7633) (16.5189, -11.7683) (16.5236, -11.7733) (16.5282, -11.7784) (16.533, -11.7835) (16.5378, -11.7887) (16.5426, -11.7939) (16.5475, -11.7991) (16.5524, -11.8043) (16.5574, -11.8096) (16.5624, -11.8149) (16.5675, -11.8203) (16.5726, -11.8257) (16.5778, -11.8311) (16.583, -11.8365) (16.5882, -11.842) (16.5935, -11.8475) (16.5989, -11.853) (16.6043, -11.8586) (16.6097, -11.8642) (16.6152, -11.8698) (16.6207, -11.8755) (16.6263, -11.8812) (16.6319, -11.8869) (16.6376, -11.8926) (16.6433, -11.8984) (16.6491, -11.9042) (16.6549, -11.91) (16.6607, -11.9159) (16.6666, -11.9218) (16.6725, -11.9277) (16.6785, -11.9336) (16.6845, -11.9395) (16.6906, -11.9455) (16.6967, -11.9515) (16.7029, -11.9576) (16.7091, -11.9636) (16.7153, -11.9697) (16.7216, -11.9758) (16.7279, -11.982) (16.7343, -11.9881) (16.7407, -11.9943) (16.7472, -12.0005) (16.7537, -12.0067) (16.7602, -12.013) (16.7668, -12.0192) (16.7735, -12.0255) (16.7801, -12.0319) (16.7869, -12.0382) (16.7936, -12.0446) (16.8004, -12.0509) (16.8073, -12.0573) (16.8142, -12.0638) (16.8211, -12.0702) (16.8281, -12.0767) (16.8351, -12.0831) (16.8421, -12.0897) (16.8492, -12.0962) (16.8564, -12.1027) (16.8636, -12.1093) (16.8708, -12.1159) (16.8781, -12.1225) (16.8854, -12.1291) (16.8927, -12.1357) (16.9001, -12.1424) (16.9075, -12.1491) (16.915, -12.1558) (16.9225, -12.1625) (16.9301, -12.1692) (16.9377, -12.1759) (16.9453, -12.1827) (16.953, -12.1895) (16.9607, -12.1963) (16.9685, -12.2031) (16.9763, -12.2099) (16.9841, -12.2168) (16.992, -12.2236) (16.9999, -12.2305) (17.0079, -12.2374) (17.0159, -12.2443) (17.0239, -12.2512) (17.032, -12.2582) (17.0401, -12.2651) (17.0483, -12.2721) (17.0565, -12.2791) (17.0647, -12.2861) (17.073, -12.2931) (17.0813, -12.3001) (17.0897, -12.3071) (17.0981, -12.3142) (17.1065, -12.3212) (17.115, -12.3283) (17.1235, -12.3354) (17.1321, -12.3425) (17.1407, -12.3496) (17.1493, -12.3568) (17.158, -12.3639) (17.1667, -12.3711) (17.1754, -12.3782) (17.1842, -12.3854) (17.1931, -12.3926) (17.2019, -12.3998) (17.2108, -12.407) (17.2198, -12.4142) (17.2288, -12.4215) (17.2378, -12.4287) (17.2469, -12.436) (17.2559, -12.4432) (17.2651, -12.4505) (17.2743, -12.4578) (17.2835, -12.4651) (17.2927, -12.4724) (17.302, -12.4797) (17.3113, -12.4871) (17.3207, -12.4944) (17.3301, -12.5017) (17.3395, -12.5091) (17.349, -12.5165) (17.3585, -12.5238) (17.3681, -12.5312) (17.3777, -12.5386) (17.3873, -12.546) (17.397, -12.5534) (17.4067, -12.5609) (17.4164, -12.5683) (17.4262, -12.5757) (17.436, -12.5832) (17.4458, -12.5906) (17.4557, -12.5981) (17.4657, -12.6055) (17.4756, -12.613) (17.4856, -12.6205) (17.4956, -12.628) (17.5057, -12.6355) (17.5158, -12.643) (17.526, -12.6505) (17.5361, -12.658) (17.5464, -12.6655) (17.5566, -12.6731) (17.5669, -12.6806) (17.5772, -12.6881) (17.5876, -12.6957) (17.598, -12.7032) (17.6084, -12.7108) (17.6189, -12.7184) (17.6294, -12.7259) (17.6399, -12.7335) (17.6505, -12.7411) (17.6611, -12.7487) (17.6718, -12.7563) (17.6825, -12.7639) (17.6932, -12.7715) (17.7039, -12.7791) (17.7147, -12.7867) (17.7256, -12.7943) (17.7364, -12.8019) (17.7473, -12.8096) (17.7583, -12.8172) (17.7692, -12.8248) (17.7802, -12.8325) (17.7913, -12.8401) (17.8023, -12.8477) (17.8112, -12.8539) (17.8179, -12.8584) (17.8224, -12.8615) (17.8246, -12.863) knots 0 0 0 0 0 0 0.00416667 0.00833333 0.0125 0.01666667 0.02083333 0.025 0.02916667 0.03333333 0.0375 0.04166667 0.04583333 0.05 0.05416667 0.05833333 0.0625 0.06666667 0.07083333 0.075 0.07916667 0.08333333 0.0875 0.09166667 0.09583333 0.1 0.10416667 0.10833333 0.1125 0.11666667 0.12083333 0.125 0.12916667 0.13333333 0.1375 0.14166667 0.14583333 0.15 0.15416667 0.15833333 0.1625 0.16666667 0.17083333 0.175 0.17916667 0.18333333 0.1875 0.19166667 0.19583333 0.2 0.20416667 0.20833333 0.2125 0.21666667 0.22083333 0.225 0.22916667 0.23333333 0.2375 0.24166667 0.24583333 0.25 0.25416667 0.25833333 0.2625 0.26666667 0.27083333 0.275 0.27916667 0.28333333 0.2875 0.29166667 0.29583333 0.3 0.30416667 0.30833333 0.3125 0.31666667 0.32083333 0.325 0.32916667 0.33333333 0.3375 0.34166667 0.34583333 0.35 0.35416667 0.35833333 0.3625 0.36666667 0.37083333 0.375 0.37916667 0.38333333 0.3875 0.39166667 0.39583333 0.4 0.40416667 0.40833333 0.4125 0.41666667 0.42083333 0.425 0.42916667 0.43333333 0.4375 0.44166667 0.44583333 0.45 0.45416667 0.45833333 0.4625 0.46666667 0.47083333 0.475 0.47916667 0.48333333 0.4875 0.49166667 0.49583333 0.5 0.50416667 0.50833333 0.5125 0.51666667 0.52083333 0.525 0.52916667 0.53333333 0.5375 0.54166667 0.54583333 0.55 0.55416667 0.55833333 0.5625 0.56666667 0.57083333 0.575 0.57916667 0.58333333 0.5875 0.59166667 0.59583333 0.6 0.60416667 0.60833333 0.6125 0.61666667 0.62083333 0.625 0.62916667 0.63333333 0.6375 0.64166667 0.64583333 0.65 0.65416667 0.65833333 0.6625 0.66666667 0.67083333 0.675 0.67916667 0.68333333 0.6875 0.69166667 0.69583333 0.7 0.70416667 0.70833333 0.7125 0.71666667 0.72083333 0.725 0.72916667 0.73333333 0.7375 0.74166667 0.74583333 0.75 0.75416667 0.75833333 0.7625 0.76666667 0.77083333 0.775 0.77916667 0.78333333 0.7875 0.79166667 0.79583333 0.8 0.80416667 0.80833333 0.8125 0.81666667 0.82083333 0.825 0.82916667 0.83333333 0.8375 0.84166667 0.84583333 0.85 0.85416667 0.85833333 0.8625 0.86666667 0.87083333 0.875 0.87916667 0.88333333 0.8875 0.89166667 0.89583333 0.9 0.90416667 0.90833333 0.9125 0.91666667 0.92083333 0.925 0.92916667 0.93333333 0.9375 0.94166667 0.94583333 0.95 0.95416667 0.95833333 0.9625 0.96666667 0.97083333 0.975 0.97916667 0.98333333 0.9875 0.99166667 0.99583333 1 1 1 1 1 1
  arc A47 (17.8246, -12.863) -> (18.6136, -12.2898) centre (0, 12.5) ccw
  spline S47 degree 5 poles (18.6136, -12.2898) (18.6128, -12.2872) (18.6113, -12.282) (18.609, -12.2743) (18.6059, -12.2639) (18.6021, -12.251) (18.5982, -12.2382) (18.5943, -12.2253) (18.5905, -12.2125) (18.5866, -12.1998) (18.5827, -12.1871) (18.5788, -12.1744) (18.5749, -12.1617) (18.571, -12.1491) (18.5671, -12.1365) (18.5632, -12.124) (18.5593, -12.1115) (18.5553, -12.099) (18.5514, -12.0866) (18.5475, -12.0742) (18.5435, -12.0618) (18.5395, -12.0495) (18.5356, -12.0372) (18.5316, -12.0249) (18.5277, -12.0127) (18.5237, -12.0005) (18.5197, -11.9884) (18.5157, -11.9762) (18.5117, -11.9642) (18.5077, -11.9521) (18.5037, -11.9401) (18.4997, -11.9281) (18.4957, -11.9162) (18.4917, -11.9043) (18.4877, -11.8925) (18.4836, -11.8806) (18.4796, -11.8689) (18.4756, -11.8571) (18.4715, -11.8454) (18.4675, -11.8337) (18.4634, -11.8221) (18.4594, -11.8105) (18.4553, -11.799) (18.4513, -11.7874) (18.4472, -11.776) (18.4431, -11.7645) (18.4391, -11.7531) (18.435, -11.7417) (18.4309, -11.7304) (18.4269, -11.7191) (18.4228, -11.7079) (18.4187, -11.6967) (18.4146, -11.6855) (18.4105, -11.6744) (18.4064, -11.6633) (18.4023, -11.6522) (18.3982, -11.6412) (18.3941, -11.6302) (18.39, -11.6193) (18.3859, -11.6084) (18.3818, -11.5975) (18.3777, -11.5867) (18.3736, -11.5759) (18.3695, -11.5652) (18.3654, -11.5545) (18.3613, -11.5438) (18.3572, -11.5332) (18.3531, -11.5226) (18.349, -11.5121) (18.3449, -11.5016) (18.3408, -11.4911) (18.3366, -11.4807) (18.3325, -11.4703) (18.3284, -11.46) (18.3243, -11.4497) (18.3202, -11.4395) (18.3161, -11.4292) (18.312, -11.4191) (18.3079, -11.409) (18.3038, -11.3989) (18.2996, -11.3888) (18.2955, -11.3788) (18.2914, -11.3689) (18.2873, -11.359) (18.2832, -11.3491) (18.2791, -11.3393) (18.275, -11.3295) (18.2709, -11.3197) (18.2668, -11.31) (18.2627, -11.3004) (18.2587, -11.2907) (18.2546, -11.2812) (18.2505, -11.2716) (18.2464, -11.2622) (18.2423, -11.2527) (18.2383, -11.2433) (18.2342, -11.234) (18.2301, -11.2247) (18.226, -11.2154) (18.222, -11.2062) (18.2179, -11.197) (18.2139, -11.1879) (18.2098, -11.1788) (18.2058, -11.1697) (18.2018, -11.1607) (18.1977, -11.1518) (18.1937, -11.1429) (18.1897, -11.134) (18.1857, -11.1252) (18.1816, -11.1165) (18.1776, -11.1077) (18.1736, -11.0991) (18.1696, -11.0904) (18.1657, -11.0818) (18.1617, -11.0733) (18.1577, -11.0648) (18.1537, -11.0564) (18.1498, -11.048) (18.1458, -11.0396) (18.1419, -11.0313) (18.1379, -11.0231) (18.134, -11.0149) (18.1301, -11.0067) (18.1262, -10.9986) (18.1223, -10.9905) (18.1184, -10.9825) (18.1145, -10.9746) (18.1106, -10.9666) (18.1068, -10.9588) (18.1029, -10.951) (18.0991, -10.9432) (18.0952, -10.9355) (18.0914, -10.9278) (18.0876, -10.9202) (18.0838, -10.9126) (18.08, -10.9051) (18.0762, -10.8976) (18.0724, -10.8902) (18.0687, -10.8828) (18.0649, -10.8755) (18.0612, -10.8683) (18.0575, -10.861) (18.0538, -10.8539) (18.0501, -10.8468) (18.0464, -10.8397) (18.0427, -10.8327) (18.039, -10.8257) (18.0354, -10.8188) (18.0318, -10.812) (18.0282, -10.8052) (18.0246, -10.7984) (18.021, -10.7918) (18.0174, -10.7851) (18.0139, -10.7785) (18.0103, -10.772) (18.0068, -10.7655) (18.0033, -10.7591) (17.9998, -10.7527) (17.9963, -10.7464) (17.9929, -10.7402) (17.9895, -10.734) (17.986, -10.7278) (17.9826, -10.7217) (17.9793, -10.7157) (17.9759, -10.7097) (17.9726, -10.7038) (17.9692, -10.6979) (17.9659, -10.6921) (17.9627, -10.6864) (17.9594, -10.6807) (17.9562, -10.6751) (17.9529, -10.6695) (17.9497, -10.664) (17.9466, -10.6585) (17.9434, -10.6531) (17.9403, -10.6478) (17.9372, -10.6425) (17.9341, -10.6373) (17.931, -10.6321) (17.928, -10.627) (17.925, -10.622) (17.922, -10.617) (17.9191, -10.6121) (17.9161, -10.6072) (17.9132, -10.6024) (17.9103, -10.5977) (17.9075, -10.593) (17.9047, -10.5884) (17.9019, -10.5839) (17.8991, -10.5794) (17.8964, -10.575) (17.8937, -10.5706) (17.891, -10.5664) (17.8883, -10.5621) (17.8857, -10.558) (17.8831, -10.5539) (17.8806, -10.5499) (17.8781, -10.5459) (17.8756, -10.542) (17.8731, -10.5382) (17.8707, -10.5344) (17.8683, -10.5308) (17.866, -10.5271) (17.8637, -10.5236) (17.8614, -10.5201) (17.8592, -10.5167) (17.857, -10.5134) (17.8548, -10.5101) (17.8527, -10.5069) (17.8506, -10.5038) (17.8485, -10.5007) (17.8465, -10.4978) (17.8446, -10.4948) (17.8427, -10.492) (17.8408, -10.4893) (17.8389, -10.4866) (17.8372, -10.484) (17.8354, -10.4814) (17.8337, -10.479) (17.8321, -10.4766) (17.8305, -10.4743) (17.8289, -10.4721) (17.8274, -10.4699) (17.826, -10.4679) (17.8246, -10.4659) (17.8232, -10.464) (17.8219, -10.4622) (17.8207, -10.4604) (17.8195, -10.4588) (17.8183, -10.4572) (17.8172, -10.4557) (17.8162, -10.4543) (17.8153, -10.453) (17.8144, -10.4518) (17.8135, -10.4506) (17.8127, -10.4496) (17.812, -10.4486) (17.8114, -10.4477) (17.8108, -10.4469) (17.8103, -10.4463) (17.8098, -10.4457) (17.8095, -10.4453) (17.8093, -10.445) (17.8092, -10.4448) (17.8091, -10.4448) knots -1 -1 -1 -1 -1 -1 -0.99583333 -0.99166667 -0.9875 -0.98333333 -0.97916667 -0.975 -0.97083333 -0.96666667 -0.9625 -0.95833333 -0.95416667 -0.95 -0.94583333 -0.94166667 -0.9375 -0.93333333 -0.92916667 -0.925 -0.92083333 -0.91666667 -0.9125 -0.90833333 -0.90416667 -0.9 -0.89583333 -0.89166667 -0.8875 -0.88333333 -0.87916667 -0.875 -0.87083333 -0.86666667 -0.8625 -0.85833333 -0.85416667 -0.85 -0.84583333 -0.84166667 -0.8375 -0.83333333 -0.82916667 -0.825 -0.82083333 -0.81666667 -0.8125 -0.80833333 -0.80416667 -0.8 -0.79583333 -0.79166667 -0.7875 -0.78333333 -0.77916667 -0.775 -0.77083333 -0.76666667 -0.7625 -0.75833333 -0.75416667 -0.75 -0.74583333 -0.74166667 -0.7375 -0.73333333 -0.72916667 -0.725 -0.72083333 -0.71666667 -0.7125 -0.70833333 -0.70416667 -0.7 -0.69583333 -0.69166667 -0.6875 -0.68333333 -0.67916667 -0.675 -0.67083333 -0.66666667 -0.6625 -0.65833333 -0.65416667 -0.65 -0.64583333 -0.64166667 -0.6375 -0.63333333 -0.62916667 -0.625 -0.62083333 -0.61666667 -0.6125 -0.60833333 -0.60416667 -0.6 -0.59583333 -0.59166667 -0.5875 -0.58333333 -0.57916667 -0.575 -0.57083333 -0.56666667 -0.5625 -0.55833333 -0.55416667 -0.55 -0.54583333 -0.54166667 -0.5375 -0.53333333 -0.52916667 -0.525 -0.52083333 -0.51666667 -0.5125 -0.50833333 -0.50416667 -0.5 -0.49583333 -0.49166667 -0.4875 -0.48333333 -0.47916667 -0.475 -0.47083333 -0.46666667 -0.4625 -0.45833333 -0.45416667 -0.45 -0.44583333 -0.44166667 -0.4375 -0.43333333 -0.42916667 -0.425 -0.42083333 -0.41666667 -0.4125 -0.40833333 -0.40416667 -0.4 -0.39583333 -0.39166667 -0.3875 -0.38333333 -0.37916667 -0.375 -0.37083333 -0.36666667 -0.3625 -0.35833333 -0.35416667 -0.35 -0.34583333 -0.34166667 -0.3375 -0.33333333 -0.32916667 -0.325 -0.32083333 -0.31666667 -0.3125 -0.30833333 -0.30416667 -0.3 -0.29583333 -0.29166667 -0.2875 -0.28333333 -0.27916667 -0.275 -0.27083333 -0.26666667 -0.2625 -0.25833333 -0.25416667 -0.25 -0.24583333 -0.24166667 -0.2375 -0.23333333 -0.22916667 -0.225 -0.22083333 -0.21666667 -0.2125 -0.20833333 -0.20416667 -0.2 -0.19583333 -0.19166667 -0.1875 -0.18333333 -0.17916667 -0.175 -0.17083333 -0.16666667 -0.1625 -0.15833333 -0.15416667 -0.15 -0.14583333 -0.14166667 -0.1375 -0.13333333 -0.12916667 -0.125 -0.12083333 -0.11666667 -0.1125 -0.10833333 -0.10416667 -0.1 -0.09583333 -0.09166667 -0.0875 -0.08333333 -0.07916667 -0.075 -0.07083333 -0.06666667 -0.0625 -0.05833333 -0.05416667 -0.05 -0.04583333 -0.04166667 -0.0375 -0.03333333 -0.02916667 -0.025 -0.02083333 -0.01666667 -0.0125 -0.00833333 -0.00416667 0 0 0 0 0 0
  line L103 (17.8091, -10.4448) -> (17.8086, -10.4441)
  line L104 (17.8086, -10.4441) -> (17.6281, -10.2115)
  arc A48 (17.6281, -10.2115) -> (18.5501, -9.4649) centre (0, 12.5) ccw
  line L105 (18.5501, -9.4649) -> (18.7401, -9.6898)
  line L106 (18.7401, -9.6898) -> (18.7406, -9.6904)